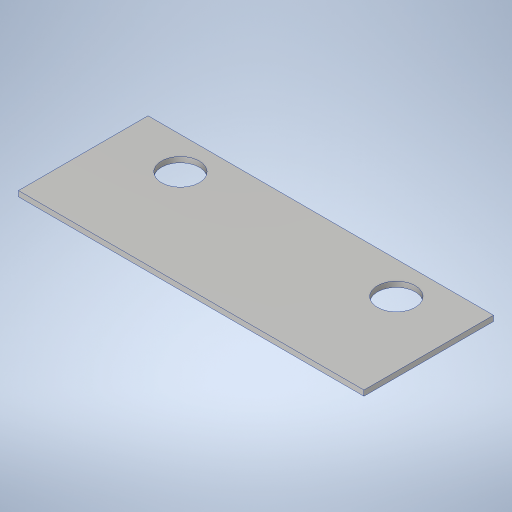
# Autodesk Inventor part: GP2-002
Saved by Autodesk Inventor 2023.4 (Build 274418000, 418)
## iProperties
Created: 2025-01-12
Part Number: GP2-002
Material: Aluminum 6061
Document SubType Name: Modeling
Designer: jmcintyr
Density: 2.7 g/cm^3
Appearance: Aluminum - Flat
Author: jmcintyr
Autodesk Inventor part; units mm, degrees
ref_plane "YZ Plane" through (0, 0, 0) normal (1, 0, 0) x (0, 1, 0)
ref_plane "XZ Plane" through (0, 0, 0) normal (0, 1, 0) x (-1, 0, 0)
ref_plane "XY Plane" through (0, 0, 0) normal (0, 0, 1) x (1, 0, 0)
sketch "Sketch1" plane through (0, 0, 0) normal (0, 1, 0) x (-1, 0, 0)
  line L0 (101.6, -38.1) -> (-101.6, -38.1)
  line L1 (-101.6, -38.1) -> (-101.6, 38.1)
  line L2 (-101.6, 38.1) -> (101.6, 38.1)
  line L3 (101.6, 38.1) -> (101.6, -38.1)
  line L4 (101.6, -38.1) -> (-101.6, 38.1) construction
  line L5 (-101.6, -38.1) -> (101.6, 38.1) construction
  point P0 (0, 0)
  dimension "d0" = 203.2
  dimension "d1" = 76.2
  constraints: 12 end point, 2 midpoint, 2 parallel, 1 horizontal, 1 perpendicular
  measures "d0" distance of L1.end L2.end
  measures "d1" distance of L0.end L1.end
extrude "Extrusion1" add sketch "Sketch1" against normal blind 3.175
sketch "Sketch2" plane through (0, 0, 0) normal (0, 1, 0) x (1, 0, 0)
  line L0 (-101.6, 38.1) -> (101.6, 38.1) construction
  line L1 (0, 38.1) -> (0, -38.1) construction
  line L2 (101.6, -38.1) -> (-101.6, -38.1) construction
  point P0 (0, 0)
  point P1 (-63.5, 19.05)
  point P2 (0, 0)
  point P3 (63.5, 19.05)
  dimension "d4" = 19.05
  dimension "d5" = 63.5
  constraints: 3 midpoint, 2 end point, 1 symmetric about line
  measures "d4" vertical distance of point (0, 0) point (-63.5, 19.05)
  measures "d5" horizontal distance of point (0, 0) point (-63.5, 19.05)
hole "Hole1" at (-63.5, 0, -19.05) at (63.5, 0, -19.05) direction (0, -1, 0) diameter 22.225 end through all
body "Solid1"
